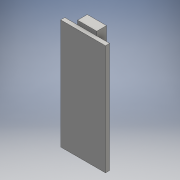
# Autodesk Inventor part: Arduino
Saved by Autodesk Inventor 2016 (Build 200138000, 138)
## iProperties
Created: 2016-04-18
Part Number: Arduino
Material: Generic
Document SubType Name: Modeling
Designer: Jarrett
Density: 1 g/cm^3
Appearance: Default
Author: Jarrett
Autodesk Inventor part; units mm, degrees
ref_plane "YZ Plane" through (0, 0, 0) normal (1, 0, 0) x (0, 1, 0)
ref_plane "XZ Plane" through (0, 0, 0) normal (0, 1, 0) x (-1, 0, 0)
ref_plane "XY Plane" through (0, 0, 0) normal (0, 0, 1) x (1, 0, 0)
sketch "Sketch1" plane through (0, 0, 0) normal (0, 1, 0) x (-1, 0, 0)
  line L0 (0, 0) -> (17.5, 0)
  line L1 (17.5, 0) -> (17.5, -43)
  line L2 (17.5, -43) -> (0, -43)
  line L3 (0, -43) -> (0, 0)
  dimension "d0" = 43
  dimension "d1" = 17.5
  constraints: 8 end point, 2 parallel, 1 horizontal, 1 perpendicular
  measures "d0" distance of L0.end L1.end
  measures "d1" distance of L0.start L0.end
extrude "Extrusion1" add sketch "Sketch1" along normal blind 1.6
sketch "Sketch2" plane through (0, 1.6, 0) normal (0, 1, 0) x (1, 0, 0)
  line L0 (-17.5, 0) -> (0, 0) projected
  line L1 (-8.75, 0) -> (-8.75, 8.3818) construction
  line L2 (-5, 7.6) -> (-12.5, 7.6)
  line L3 (-12.5, 7.6) -> (-12.5, -1.6)
  line L4 (-12.5, -1.6) -> (-5, -1.6)
  line L5 (-5, -1.6) -> (-5, 7.6)
  line L6 (-5, 7.6) -> (-12.5, -1.6) construction
  line L7 (-12.5, 7.6) -> (-5, -1.6) construction
  point P0 (-8.75, 3)
  dimension "d4" = 9.2
  dimension "d5" = 7.5
  dimension "d6" = 1.6
  constraints: 14 end point, 3 midpoint, 2 parallel, 1 horizontal, 1 perpendicular, 1 point on line, 1 vertical
  measures "d4" distance of L2.end L3.end
  measures "d5" distance of L3.end L4.end
  measures "d6" distance between parallel lines of L0 L4
extrude "Extrusion2" add sketch "Sketch2" along normal blind 3.8
body "Solid1"
